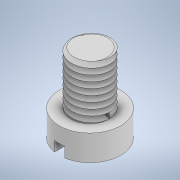
# Autodesk Inventor part: Винт 5x8
Saved by Autodesk Inventor 2020 (Build 240168000, 168)
## iProperties
Created: 2021-04-26
Part Number: Винт 5x8
Material: Типовые
Document SubType Name: Modeling
Designer: lbfas
Density: 1 g/cm^3
Appearance: По умолчанию
Author: lbfas
Autodesk Inventor part; units mm, degrees
ref_plane "YZ Plane" through (0, 0, 0) normal (1, 0, 0) x (0, 1, 0)
ref_plane "XZ Plane" through (0, 0, 0) normal (0, 1, 0) x (-1, 0, 0)
ref_plane "XY Plane" through (0, 0, 0) normal (0, 0, 1) x (1, 0, 0)
sketch "Эскиз1" plane through (0, 0, 0) normal (0, 1, 0) x (-1, 0, 0)
  circle A0 centre (0, 0) radius 6
  dimension "d0" = 12
  constraints: 1 centre point, 1 coincident
  measures "d0" diameter of A0
extrude "Выдавливание1" add sketch "Эскиз1" along normal blind 5
sketch "Эскиз2" plane through (0, 5, 0) normal (0, 1, 0) x (1, 0, 0)
  circle A0 centre (0, 0) radius 3.75
  dimension "d3" = 7.5
  constraints: 1 centre point, 1 coincident
  measures "d3" diameter of A0
extrude "Выдавливание2" add sketch "Эскиз2" along normal blind 10.5
sketch "Эскиз3" plane through (0, 0, 0) normal (0, 0, 1) x (1, 0, 0)
  line L0 (3.75, 5) -> (3.75, 15.5) projected
  line L1 (3.75, 5.5775) -> (2.7497, 5.5775)
  line L2 (6, 5) -> (-6, 5) projected
  line L3 (2.7497, 5.5775) -> (3.75, 5)
  line L4 (3.75, 5.5775) -> (3.75, 5)
  line L5 (2.7497, 5.5775) -> (3.75, 6.155)
  line L6 (3.75, 5.5775) -> (3.75, 6.155)
  point P0 (0, 0)
  dimension "d7" = 1.155
  dimension "d8" = 30
  constraints: 10 end point, 1 symmetric about line, 1 vertical
  measures "d7" distance of L0.start L1.end
  measures "d8" angle of L3 L1
coil "Пружина1" sketch "Эскиз3" operation cut axis through (0, 5, 0) along (0, 1, 0) pitch 1.155 turns 12.987013 hand left
sketch "Эскиз4" plane through (0, 0, 0) normal (0, -1, 0) x (1, 0, 0)
  line L0 (1, 0) -> (1, 5.9161)
  circle A0 centre (0, 0) radius 6 projected
  line L1 (1, 0) -> (1, -5.9161)
  line L2 (-1, 0) -> (-1, 5.9161)
  line L3 (-1, 0) -> (-1, -5.9161)
  constraints: 8 end point, 2 other
extrude "Выдавливание3" cut sketch "Эскиз4" against normal blind 2 contours L1 A0 L3 L2 L0
